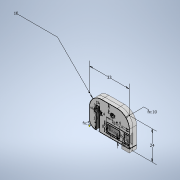
# Autodesk Inventor part: Front
Saved by Autodesk Inventor 2020 (Build 240168000, 168)
## iProperties
Created: 2022-09-30
Part Number: Front
Material: Generic
Document SubType Name: Modeling
Designer: jsp534
Density: 1 g/cm^3
Appearance: Default
Author: jsp534
Autodesk Inventor part; units mm, degrees
ref_plane "YZ Plane" through (0, 0, 0) normal (1, 0, 0) x (0, 1, 0)
ref_plane "XZ Plane" through (0, 0, 0) normal (0, 1, 0) x (-1, 0, 0)
ref_plane "XY Plane" through (0, 0, 0) normal (0, 0, 1) x (1, 0, 0)
sketch "Sketch1" plane through (0, 0, 0) normal (0, 0, 1) x (1, 0, 0)
  line L0 (5, 0) -> (5.475, 0)
  line L1 (33, 0) -> (33, 14)
  line L2 (23, 24) -> (10, 24)
  line L3 (0, 14) -> (0, 5)
  line L4 (5.475, 0) -> (5.475, 12.6)
  line L5 (5.475, 12.6) -> (4, 12.6)
  line L6 (4, 12.6) -> (4, 15)
  line L7 (4, 15) -> (5.475, 15)
  line L8 (5.475, 15) -> (5.475, 18)
  line L9 (5.475, 18) -> (8.475, 18)
  line L10 (8.475, 18) -> (8.475, 15)
  line L11 (8.475, 15) -> (9.95, 15)
  line L12 (9.95, 15) -> (9.95, 12.6)
  line L13 (9.95, 12.6) -> (8.475, 12.6)
  line L14 (8.475, 12.6) -> (8.475, 0)
  circle A0 centre (19, 17) radius 1.6
  line L15 (5.475, 0) -> (8.475, 0) construction
  line L16 (8.475, 0) -> (33, 0)
  line L17 (33, 2) -> (14.1, 2)
  line L18 (14.1, 2) -> (14.1, 6.05)
  line L19 (14.1, 10.1) -> (33, 10.1)
  line L20 (33, 10.1) -> (33, 2)
  line L21 (33, 9.1) -> (28.7, 9.1)
  line L22 (28.7, 9.1) -> (28.7, 6.05)
  line L23 (28.7, 3) -> (33, 3)
  line L24 (33, 3) -> (33, 9.1)
  line L25 (14.9, 8.85) -> (25, 8.85)
  line L26 (25, 8.85) -> (25, 3.25)
  line L27 (25, 3.25) -> (14.9, 3.25)
  line L28 (14.9, 3.25) -> (14.9, 6.05)
  line L29 (14.1, 6.05) -> (33, 6.05) construction
  line L30 (14.9, 6.05) -> (14.9, 8.85)
  line L31 (28.7, 6.05) -> (28.7, 3)
  line L32 (14.1, 6.05) -> (14.1, 10.1)
  arc A1 (10, 24) -> (0, 14) centre (10, 14) ccw
  arc A2 (33, 14) -> (23, 24) centre (23, 14) ccw
  arc A3 (0, 5) -> (5, 0) centre (5, 5) ccw
  point P0 (0, 0)
  point P1 (33, 24)
  point P2 (0, 24)
  dimension "totalWidth" = 33
  dimension "totalHeight" = 24
  dimension "edgeToNut" = 4
  dimension "boltHoleWidth" = 3
  dimension "nutSlotEndOffset" = 3
  dimension "boltHoleLength" = 18
  dimension "nutSlotDepth" = 2.4
  dimension "nutSlotWidth" = 5.95
  dimension "boltVertOffset" = 7
  dimension "boltDiameter" = 3.2
  dimension "boltHorizOffset" = 14
  dimension "IRSensorLength" = 18.9
  dimension "IRSensorHeight" = 8.1
  dimension "IRSensorVertOffset" = 2
  dimension "IRModuleHeight" = 5.6
  dimension "IRModuleLength" = 10.1
  dimension "moduleConnectorGap" = 3.7
  dimension "connectorHeight" = 6.1
  dimension "connectorWidth" = 4.3
  dimension "topFillet" = 10
  dimension "d20" = 10
  dimension "d21" = 5
  constraints: 66 end point, 19 point on line, 15 perpendicular, 13 parallel, 6 horizontal, 6 point on circle, 6 tangent, 4 centre point, 4 collinear, 1 midpoint, 1 vertical
  measures "totalWidth" distance of point (0, 24) point (33, 24)
  measures "totalHeight" distance of point (33, 24) L1.start
  measures "edgeToNut" distance between parallel lines of L6 L3
  measures "boltHoleWidth" distance of L8.end L9.end
  measures "nutSlotEndOffset" distance of L7.end L8.end
  measures "boltHoleLength" distance between parallel lines of L0 L9
  measures "nutSlotDepth" distance of L11.end L12.end
  measures "nutSlotWidth" distance between parallel lines of L12 L6
  measures "boltVertOffset" distance from line of L2 A0.centre
  measures "boltDiameter" diameter of A0
  measures "boltHorizOffset" distance from line of L1 A0.centre
  measures "IRSensorLength" distance of L19.start L19.end
  measures "IRSensorHeight" distance of L17.end L19.start
  measures "IRSensorVertOffset" distance between parallel lines of L17 L16
  measures "IRModuleHeight" distance between parallel lines of L27 L25
  measures "IRModuleLength" distance of L26.end L27.end
  measures "moduleConnectorGap" distance between parallel lines of L22 L26
  measures "connectorHeight" distance between parallel lines of L21 L23
  measures "connectorWidth" distance of L23.start L23.end
  measures "topFillet" radius of A1
  measures "d20" radius of A2
  measures "d21" radius of A3
extrude "Extrusion1" add sketch "Sketch1" against normal blind 3 contours A3 L3 A1 L2 A2 L1 L19 L32 L18 L17 L16 L14 L13 L12 L11 L10 L9 L8 L7 L6 L5 L4 L0 | L1 L21 L22 L31 L23 L17 L18 L32 L19
fillet "Fillet1" radius 1 2 edges at (5.475, 18, -1.5) (8.475, 18, -1.5)
fillet "Fillet2" radius 0.5 2 edges at (4, 12.6, -1.5) (9.95, 12.6, -1.5)
extrude "Extrusion2" add sketch "Sketch1" against normal blind 3 from surface at -3 separate body contours A3 L3 A1 L2 A2 L1 L19 L32 L18 L17 L16 L14 L13 L12 L11 L10 L9 L8 L7 L6 L5 L4 L0 | L1 L21 L22 L31 L23 L17 L18 L32 L19 | L1 L23 L31 L22 L21 | L25 L26 L27 L28 L30
sketch "Sketch2" plane through (33, 0, -6) normal (0, 0, -1) x (-1, 0, 0)
  circle A0 centre (14, 17) radius 1.6 projected
  line L0 (15.6454, 19.85) -> (17.2909, 17)
  line L1 (17.2909, 17) -> (15.6454, 14.15)
  line L2 (15.6454, 14.15) -> (12.3546, 14.15)
  line L3 (12.3546, 14.15) -> (10.7091, 17)
  line L4 (10.7091, 17) -> (12.3546, 19.85)
  line L5 (12.3546, 19.85) -> (15.6454, 19.85)
  line L6 (23, 24) -> (10, 24) projected
  point P0 (33, 0)
  dimension "nutSlotDiameter" = 5.7
  constraints: 12 end point, 1 coincident, 1 parallel, 13 other
  measures "nutSlotDiameter" distance between parallel lines of L1 L4
extrude "Extrusion3" cut sketch "Sketch2" against normal blind 1.5 bodies 2
sketch "Sketch3" plane through (8.475, 0, 0) normal (0, -1, 0) x (1, 0, 0)
  line L0 (24.525, -6) -> (0, -6) projected
  line L1 (24.525, -6) -> (18.525, -6)
  line L2 (18.525, -6) -> (18.525, 0)
  line L3 (18.525, 0) -> (24.525, 0)
  line L4 (24.525, 0) -> (24.525, -6)
  line L5 (24.525, -6) -> (24.525, -3) projected
  line L6 (24.525, -3) -> (18.525, -3)
  line L7 (24.525, -3) -> (0, -3) projected
  point P0 (-8.475, 0)
  dimension "d31" = 6
  dimension "d32" = 6
  constraints: 10 end point, 2 parallel, 1 horizontal, 1 midpoint, 1 perpendicular, 1 point on line
  measures "d31" distance between parallel lines of L2 L4
  measures "d32" distance between parallel lines of L0 L3
extrude "Extrusion4" add sketch "Sketch3" along normal blind 3 contours L6 L2 L3 L4 bodies 1
extrude "Extrusion5" add sketch "Sketch3" along normal blind 3 contours L0 L2 L6 L4 bodies 2
sketch "Sketch4" plane through (10, 24, -3) normal (0, 0, 1) x (1, 0, 0)
  line L0 (4.1, -13.9) -> (23, -13.9) projected
  line L1 (23, -13.9) -> (23, -22) projected
  line L2 (23, -22) -> (4.1, -22) projected
  line L3 (4.1, -22) -> (4.1, -17.95) projected
  line L4 (4.1, -17.95) -> (4.1, -13.9) projected
  point P0 (-10, -24)
extrude "Extrusion6" cut sketch "Sketch4" along normal blind 1 bodies 1
fillet "Fillet3" radius 1 2 edges at (5.475, 18, -4.5) (8.475, 18, -4.5)
fillet "Fillet4" radius 0.5 2 edges at (9.95, 12.6, -4.5) (4, 12.6, -4.5)
equation "\"d20\" = topFillet"
equation "\"d21\" = 0.5 * topFillet"
equation "\"d29\" = 0.5 * perspexThickness"
equation "\"d31\" = 2 * perspexThickness"
equation "\"d32\" = 2 * perspexThickness"
equation "\"d33\" = perspexThickness"
equation "\"d35\" = perspexThickness"
equation "\"perspexThickness\" = 3"
